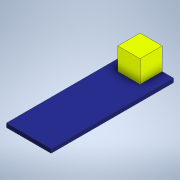
# Autodesk Inventor part: WaterSensor
Saved by Autodesk Inventor 2021 (Build 250183000, 183)
## iProperties
Created: 2021-01-19
Part Number: WaterSensor
Material: Generic
Document SubType Name: Modeling
Designer: Jayan
Density: 1 g/cm^3
Appearance: Default
Author: Jayan
Autodesk Inventor part; units mm, degrees
ref_plane "YZ Plane" through (0, 0, 0) normal (1, 0, 0) x (0, 1, 0)
ref_plane "XZ Plane" through (0, 0, 0) normal (0, 1, 0) x (-1, 0, 0)
ref_plane "XY Plane" through (0, 0, 0) normal (0, 0, 1) x (1, 0, 0)
sketch "Sketch1" plane through (0, 0, 0) normal (0, 1, 0) x (-1, 0, 0)
  line L0 (0, 0) -> (25.4, 0)
  line L1 (25.4, 0) -> (25.4, -69.85)
  line L2 (25.4, -69.85) -> (0, -69.85)
  line L3 (0, -69.85) -> (0, 0)
  dimension "d0" = 25.4
  dimension "d1" = 69.85
  constraints: 8 end point, 2 parallel, 1 horizontal, 1 perpendicular
  measures "d0" distance of L1.end L2.end
  measures "d1" distance of L0.end L1.end
extrude "Extrusion1" add sketch "Sketch1" along normal blind 2.3813
sketch "Sketch2" plane through (0, 2.3813, 0) normal (0, 1, 0) x (1, 0, 0)
  line L0 (0, 69.85) -> (-25.4, 69.85) projected
  line L1 (0, 69.85) -> (-6.35, 69.85)
  line L2 (-6.35, 69.85) -> (-19.05, 69.85)
  line L3 (-19.05, 69.85) -> (-19.05, 57.15)
  line L4 (-19.05, 57.15) -> (-6.35, 57.15)
  line L5 (-6.35, 57.15) -> (-6.35, 69.85)
  point P0 (0, 0)
  dimension "d4" = 6.35
  dimension "d5" = 12.7
  dimension "d6" = 12.7
  constraints: 10 end point, 2 parallel, 1 horizontal, 1 perpendicular, 1 point on line
  measures "d4" distance of L0.start L1.end
  measures "d5" distance of L4.end L3.end
  measures "d6" distance of L3.end L2.end
extrude "Extrusion2" add sketch "Sketch2" along normal blind 12.7
body "Solid1"
